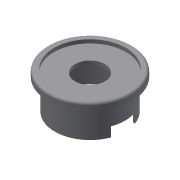
# Autodesk Inventor part: Tapa_superior_carcasa
Saved by Autodesk Inventor 2013 SP2 (Build 170200200, 200)
## iProperties
Created: 2014-01-13
Part Number: Tapa_superior_carcasa
Material: Generic
Document SubType Name: Modeling
Designer: Koky
Density: 1 g/cm^3
Author: Koky
Autodesk Inventor part; units mm, degrees
ref_plane "XZ Plane" through (0, 0, 0) normal (0, 1, 0) x (-1, 0, 0)
ref_plane "XY Plane" through (0, 0, 0) normal (0, 0, 1) x (1, 0, 0)
sketch "Sketch1" plane through (0, 0, 0) normal (0, 0, 1) x (1, 0, 0)
  circle A0 centre (0, 0) radius 35
  dimension "d0" = 70
  constraints: 1 centre point, 1 coincident
  measures "d0" diameter of A0
extrude "Extrusion1" add sketch "Sketch1" along normal blind 6
sketch "Sketch2" plane through (0, 0, 6) normal (0, 0, 1) x (1, 0, 0)
  circle A0 centre (0, 0) radius 35 projected
  circle A1 centre (0, 0) radius 30
  dimension "d3" = 60
  constraints: 1 centre point, 1 coincident
  measures "d3" diameter of A1
extrude "Extrusion2" cut sketch "Sketch2" against normal blind 3 contours A1
sketch "Sketch3" plane through (0, 0, 0) normal (0, 0, -1) x (-1, 0, 0)
  circle A0 centre (0, 0) radius 35 projected
  circle A1 centre (0, 0) radius 29.35
  circle A2 centre (0, 0) radius 27.85
  dimension "d6" = 58.7
  dimension "d7" = 55.7
  constraints: 2 centre point, 2 coincident
  measures "d6" diameter of A1
  measures "d7" diameter of A2
extrude "Extrusion3" add sketch "Sketch3" along normal blind 25 contours A1
fillet "Fillet1" radius 2 1 edges at (-35, 0, 6)
sketch "Sketch4" plane through (0, 0, 3) normal (0, 0, 1) x (1, 0, 0)
  circle A0 centre (0, 0) radius 30 projected
  circle A1 centre (0, 0) radius 12.5
  dimension "d11" = 25
  constraints: 1 centre point, 1 coincident
  measures "d11" diameter of A1
extrude "Extrusion4" cut sketch "Sketch4" against normal blind 10 contours A1
ref_plane "Work Plane1" through (29.85, 0, 0) normal (1, 0, 0) x (0, 1, 0)
sketch "Sketch5" plane through (29.85, 0, 0) normal (1, 0, 0) x (0, 1, 0)
  line L0 (-10, -17) -> (10, -17)
  line L1 (10, -17) -> (10, -28.5985)
  line L2 (10, -28.5985) -> (-10, -28.5985)
  line L3 (-10, -28.5985) -> (-10, -17)
  line L4 (0, -31.2) -> (0, 12.2) projected
  line L5 (0, 0) -> (-49, 0)
  dimension "d15" = 20
  dimension "d17" = 17
  constraints: 10 end point, 2 parallel, 2 perpendicular, 1 horizontal, 1 other
  measures "d15" distance of L0.start L0.end
  measures "d17" distance between parallel lines of L5 L0
extrude "Extrusion5" cut sketch "Sketch5" against normal blind 10
body "Solid1"
